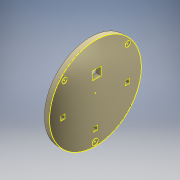
# Autodesk Inventor part: ET16
Saved by Autodesk Inventor 2016 (Build 200138000, 138)
## iProperties
Created: 2016-03-28
Part Number: ET16
Material: Genérico
Document SubType Name: Modeling
Designer: Usuario1
Density: 1 g/cm^3
Appearance: Valor por defecto
Author: Usuario1
Autodesk Inventor part; units mm, degrees
ref_plane "YZ Plane" through (0, 0, 0) normal (1, 0, 0) x (0, 1, 0)
ref_plane "XZ Plane" through (0, 0, 0) normal (0, 1, 0) x (-1, 0, 0)
ref_plane "XY Plane" through (0, 0, 0) normal (0, 0, 1) x (1, 0, 0)
sketch "Boceto1" plane through (0, 0, 0) normal (1, 0, 0) x (0, 1, 0)
  circle A0 centre (0, 0) radius 1.15
  circle A1 centre (0, 0) radius 1.0926
  constraints: 2 centre point
extrude "Extrusión1" add sketch "Boceto1" along normal blind 0.12 contours A1
sketch "Boceto2" plane through (0.12, 0, 0) normal (1, 0, 0) x (0, 0, -1)
  circle A0 centre (0, 0) radius 1.0926
  line L0 (0.79, 0.14) -> (0.51, 0.14)
  line L1 (0.51, 0.14) -> (0.51, -0.14)
  line L2 (0.51, -0.14) -> (0.79, -0.14)
  line L3 (0.79, -0.14) -> (0.79, 0.14)
  line L4 (-0.51, 0.14) -> (-0.79, 0.14)
  line L5 (-0.79, 0.14) -> (-0.79, -0.14)
  line L6 (-0.79, -0.14) -> (-0.51, -0.14)
  line L7 (-0.51, -0.14) -> (-0.51, 0.14)
  constraints: 16 end point, 1 centre point
extrude "Extrusión2" add sketch "Boceto2" against normal blind 0.25 contours L3 L2 L1 L0 | L7 L6 L5 L4
sketch "Boceto3" plane through (0.12, 0, 0) normal (1, 0, 0) x (0, 0, -1)
  circle A0 centre (0, 0) radius 1.0926
  circle A1 centre (-0.389, 0.0377) radius 0.6841
  circle A2 centre (-0.6284, -0.7346) radius 0.0625
  circle A3 centre (-0.6284, 0.7722) radius 0.0625
  line L0 (-0.2217, -0.7829) -> (-0.172, -0.9902)
  line L1 (0.4827, -0.8628) -> (0.4482, -0.6469)
  arc A4 (0.4827, -0.8628) -> (-0.172, -0.9902) centre (0.3728, -2.0444) ccw
  arc A5 (-0.2217, -0.7829) -> (-0.0098, -0.6943) centre (-0.3611, -0.1519) ccw
  arc A6 (0.2046, -0.6494) -> (-0.0098, -0.6943) centre (0.1354, -0.8536) ccw
  arc A7 (0.2046, -0.6494) -> (0.4482, -0.6469) centre (0.3201, -0.0382) ccw
  line L2 (0.623, 0.1405) -> (0.623, -0.1283)
  line L3 (0.8433, -0.1283) -> (0.8433, 0.1405)
  arc A8 (0.8433, 0.1405) -> (0.623, 0.1405) centre (0.7332, 0.1405) ccw
  arc A9 (0.623, -0.1283) -> (0.8433, -0.1283) centre (0.7332, -0.1283) ccw
  circle A10 centre (1.0028, -0.0033) radius 0.0698
  line L4 (0.48, 0.6571) -> (0.5054, 0.8687)
  line L5 (-0.1528, 0.9768) -> (-0.1954, 0.7624)
  arc A11 (-0.1528, 0.9768) -> (0.5054, 0.8687) centre (0.3609, 2.0465) ccw
  arc A12 (0.48, 0.6571) -> (0.2505, 0.6476) centre (0.3914, 0.0169) ccw
  arc A13 (0.0338, 0.6801) -> (0.2505, 0.6476) centre (0.1696, 0.8475) ccw
  arc A14 (0.0338, 0.6801) -> (-0.1954, 0.7624) centre (-0.2869, 0.147) ccw
  line L6 (-0.389, 0.0377) -> (-0.489, 0.0377)
  line L7 (-0.489, 0.0377) -> (-0.489, 0.1377)
  line L8 (-0.489, 0.1377) -> (-0.289, 0.1377)
  line L9 (-0.289, 0.1377) -> (-0.289, -0.0623)
  line L10 (-0.289, -0.0623) -> (-0.489, -0.0623)
  line L11 (-0.489, -0.0623) -> (-0.489, 0.0377)
  line L12 (0.6832, 0.0061) -> (0.6832, 0.0561)
  line L13 (0.6832, 0.0561) -> (0.7832, 0.0561)
  line L14 (0.7832, 0.0561) -> (0.7832, -0.0439)
  line L15 (0.7832, -0.0439) -> (0.6832, -0.0439)
  line L16 (0.6832, -0.0439) -> (0.6832, 0.0061)
  line L17 (0.103, 0.813) -> (0.103, 0.713)
  line L18 (0.103, 0.713) -> (0.203, 0.713)
  line L19 (0.203, 0.713) -> (0.203, 0.813)
  line L20 (0.203, 0.813) -> (0.103, 0.813)
  line L21 (0.0653, -0.725) -> (0.0653, -0.825)
  line L22 (0.0653, -0.825) -> (0.1653, -0.825)
  line L23 (0.1653, -0.825) -> (0.1653, -0.725)
  line L24 (0.1653, -0.725) -> (0.0653, -0.725)
  dimension "d6" = 0.1
  dimension "d7" = 0.1
  dimension "d8" = 0.2
  dimension "d9" = 0.2
  dimension "d10" = 0.2
  dimension "d12" = 0.05
  dimension "d13" = 0.1
  dimension "d14" = 0.1
  dimension "d15" = 0.1
  dimension "d16" = 0.1
  dimension "d17" = 0.1
  dimension "d18" = 0.1
  dimension "d19" = 0.1
  dimension "d20" = 0.1
  dimension "d21" = 0.1
  constraints: 50 end point, 20 point on circle, 15 centre point, 9 perpendicular, 2 point on line, 2 vertical, 1 collinear, 1 horizontal
  measures "d6" distance of L6.start L6.end
  measures "d7" distance of L6.end L7.end
  measures "d8" distance of L7.end L8.end
  measures "d9" distance of L8.end L9.end
  measures "d10" distance of L9.end L10.end
  measures "d12" distance of L12.start L12.end
  measures "d13" distance of L12.end L13.end
  measures "d14" distance of L13.end L14.end
  measures "d15" distance of L14.end L15.end
  measures "d16" distance of L17.start L17.end
  measures "d17" distance of L17.end L18.end
  measures "d18" distance of L18.end L19.end
  measures "d19" distance of L21.start L21.end
  measures "d20" distance of L21.end L22.end
  measures "d21" distance of L22.end L23.end
extrude "Extrusión3" cut sketch "Boceto3" against normal blind 0.25 contours L7 L8 L9 L10 L11 | L12 L13 L14 L15 L16 | L20 L19 L18 L17 | L24 L23 L22 L21
sketch "Boceto4" plane through (0.12, 0, 0) normal (1, 0, 0) x (0, 0, -1)
  circle A0 centre (0, 0) radius 1.0926
  circle A1 centre (-0.389, 0.0377) radius 0.6841
  circle A2 centre (-0.6284, -0.7346) radius 0.0625
  circle A3 centre (-0.6284, 0.7722) radius 0.0625
  line L0 (-0.2217, -0.7829) -> (-0.172, -0.9902)
  line L1 (0.4827, -0.8628) -> (0.4482, -0.6469)
  arc A4 (0.4827, -0.8628) -> (-0.172, -0.9902) centre (0.3728, -2.0444) ccw
  arc A5 (-0.2217, -0.7829) -> (-0.0098, -0.6943) centre (-0.3611, -0.1519) ccw
  arc A6 (0.2046, -0.6494) -> (-0.0098, -0.6943) centre (0.1354, -0.8536) ccw
  arc A7 (0.2046, -0.6494) -> (0.4482, -0.6469) centre (0.3201, -0.0382) ccw
  line L2 (0.623, 0.1405) -> (0.623, -0.1283)
  line L3 (0.8433, -0.1283) -> (0.8433, 0.1405)
  arc A8 (0.8433, 0.1405) -> (0.623, 0.1405) centre (0.7332, 0.1405) ccw
  arc A9 (0.623, -0.1283) -> (0.8433, -0.1283) centre (0.7332, -0.1283) ccw
  circle A10 centre (1.0028, -0.0033) radius 0.0698
  line L4 (0.48, 0.6571) -> (0.5054, 0.8687)
  line L5 (-0.1528, 0.9768) -> (-0.1954, 0.7624)
  arc A11 (-0.1528, 0.9768) -> (0.5054, 0.8687) centre (0.3609, 2.0465) ccw
  arc A12 (0.48, 0.6571) -> (0.2505, 0.6476) centre (0.3914, 0.0169) ccw
  arc A13 (0.0338, 0.6801) -> (0.2505, 0.6476) centre (0.1696, 0.8475) ccw
  arc A14 (0.0338, 0.6801) -> (-0.1954, 0.7624) centre (-0.2869, 0.147) ccw
  point P0 (0, 0)
  constraints: 20 point on circle, 15 centre point, 12 end point
extrude "Extrusión4" cut sketch "Boceto4" against normal blind 0.02 contours A2 | A3 | A10
sketch "Boceto6" plane through (0.12, 0, 0) normal (1, 0, 0) x (0, 0, -1)
  circle A0 centre (-0.6284, 0.7722) radius 0.0625 projected
  circle A1 centre (-0.6284, -0.7346) radius 0.0625 projected
  circle A2 centre (1.0028, -0.0033) radius 0.0698 projected
  line L0 (0.203, 0.713) -> (0.103, 0.713) projected
  line L1 (0.103, 0.713) -> (0.103, 0.813) projected
  line L2 (0.103, 0.813) -> (0.203, 0.813) projected
  line L3 (0.203, 0.813) -> (0.203, 0.713) projected
  line L4 (0.7832, -0.0439) -> (0.6832, -0.0439) projected
  line L5 (0.6832, -0.0439) -> (0.6832, 0.0561) projected
  line L6 (0.6832, 0.0561) -> (0.7832, 0.0561) projected
  line L7 (0.7832, 0.0561) -> (0.7832, -0.0439) projected
  line L8 (0.1653, -0.825) -> (0.0653, -0.825) projected
  line L9 (0.0653, -0.825) -> (0.0653, -0.725) projected
  line L10 (0.0653, -0.725) -> (0.1653, -0.725) projected
  line L11 (0.1653, -0.725) -> (0.1653, -0.825) projected
  line L12 (-0.289, -0.0623) -> (-0.489, -0.0623) projected
  line L13 (-0.489, -0.0623) -> (-0.489, 0.1377) projected
  line L14 (-0.489, 0.1377) -> (-0.289, 0.1377) projected
  line L15 (-0.289, 0.1377) -> (-0.289, -0.0623) projected
  circle A3 centre (0, 0) radius 1.0926 projected
